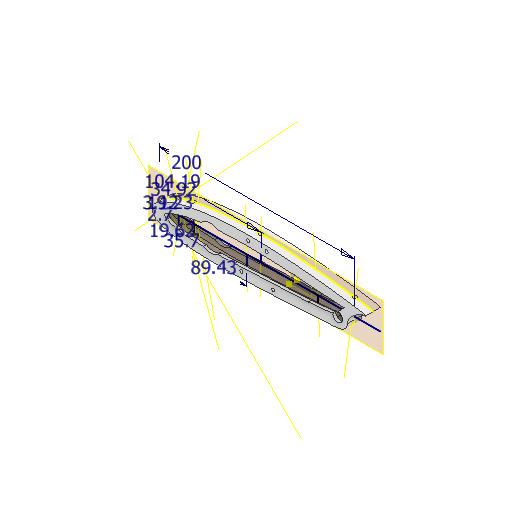
# Autodesk Inventor part: 4P.01.01.11-TW-v1-WingRibWFlapSingle
Saved by Autodesk Inventor 2025.2 (Build 292293000, 293)
## iProperties
Created: 2025-01-11
Part Number: 4P.01.01.11-TW-v1-WingRibWFlapSingle
Material: Polystyrene
Document SubType Name: Modeling
Designer: thoma
Density: 1.021 g/cm^3
Appearance: Smooth - White
Author: thoma
Autodesk Inventor part; units mm, degrees
(part 1 of 2)
ref_plane "YZ Plane" through (0, 0, 0) normal (1, 0, 0) x (0, 1, 0)
ref_plane "XZ Plane" through (0, 0, 0) normal (0, 1, 0) x (-1, 0, 0)
ref_plane "XY Plane" through (0, 0, 0) normal (0, 0, 1) x (1, 0, 0)
sketch "Sketch3" plane through (0, 0, 0) normal (0, 0, 1) x (1, 0, 0)
  line L0 (59.6953, 14.884) -> (59.6953, -12.7998) construction
  spline S0 degree 4 poles (78.1029, 11.0141) (75.5683, 12.9654) (71.7145, 13.0272) (66.8099, 13.9036) (60.7685, 14.7338) (56.2959, 15.3578) (51.7728, 15.9509) (47.2242, 16.5426) (42.6244, 17.1111) (37.9974, 17.6651) (33.3378, 18.1987) (28.6546, 18.7114) (23.9504, 19.2026) (19.2309, 19.6699) (14.5002, 20.1135) (9.7632, 20.5291) (5.025, 20.9191) (0.2903, 21.2792) (-4.4372, 21.6095) (-9.151, 21.9092) (-13.8524, 22.1766) (-18.5268, 22.4102) (-23.2002, 22.6105) (-27.8558, 22.7627) (-32.4748, 22.8704) (-37.0553, 22.9312) (-41.5904, 22.9454) (-46.0738, 22.9127) (-50.5027, 22.8323) (-54.8678, 22.7052) (-59.1755, 22.5324) (-63.394, 22.3084) (-67.5752, 22.0492) (-71.5451, 21.7209) (-75.7777, 21.4072) (-79.04, 20.9063) (-83.4863, 20.5541) (-87.0067, 20.037) (-90.7113, 19.5168) (-94.2172, 18.9459) (-97.6363, 18.3426) (-100.9342, 17.7015) (-104.1216, 17.0263) (-107.1909, 16.3187) (-110.1396, 15.5797) (-112.9656, 14.8117) (-115.6652, 14.0172) (-118.2357, 13.1965) (-120.6759, 12.3541) (-122.9817, 11.4895) (-125.1529, 10.6071) (-127.1857, 9.7065) (-129.0794, 8.7914) (-130.8324, 7.8633) (-132.4429, 6.923) (-133.9096, 5.9737) (-135.2322, 5.016) (-136.4083, 4.0508) (-137.4392, 3.0816) (-138.3215, 2.1025) (-139.0592, 1.1321) (-139.6407, 0.1249) (-140.106, -0.8362) (-140.3589, -2.0477) (-140.602, -2.598) (-140.1166, -5.4607) (-140.0539, -5.4622) (-139.4639, -6.7645) (-138.8842, -7.4979) (-138.1173, -8.3934) (-137.2199, -9.1877) (-136.1721, -9.9852) (-134.9893, -10.738) (-133.6669, -11.4655) (-132.2091, -12.1599) (-130.6156, -12.8245) (-128.8897, -13.4579) (-127.0312, -14.0591) (-125.0439, -14.6296) (-122.9287, -15.1678) (-120.6879, -15.6738) (-118.3241, -16.1476) (-115.8396, -16.5892) (-113.2366, -16.9984) (-110.5176, -17.3742) (-107.6861, -17.7183) (-104.7439, -18.0297) (-101.6943, -18.3095) (-98.5398, -18.5568) (-95.2843, -18.7732) (-91.9297, -18.9579) (-88.48, -19.1131) (-84.9381, -19.2376) (-81.3071, -19.3341) (-77.5906, -19.4015) (-73.7915, -19.4421) (-69.9139, -19.4561) (-65.961, -19.445) (-61.9362, -19.4102) (-57.8434, -19.3518) (-53.6861, -19.2727) (-49.4679, -19.1731) (-45.1932, -19.0538) (-40.8649, -18.9183) (-36.4879, -18.766) (-32.0649, -18.5992) (-27.598, -18.4192) (-23.0941, -18.227) (-18.5434, -18.0273) (-13.9382, -17.8076) (-9.3141, -17.5719) (-4.666, -17.3195) (-0.0002, -17.052) (4.6675, -16.7728) (9.3655, -16.4759) (14.0236, -16.1832) (19.545, -15.7815) (23.3079, -15.6072) (27.1098, -15.1781) (28.8959, -15.0599) knots 0 0 0 0 0 0.024672 0.034555 0.0445 0.054495 0.064543 0.074632 0.084755 0.094911 0.105094 0.115299 0.125521 0.135755 0.145995 0.156237 0.166475 0.176705 0.186921 0.197118 0.207299 0.217463 0.227605 0.23772 0.247796 0.257824 0.267798 0.277713 0.287563 0.297345 0.307053 0.31668 0.326224 0.335555 0.344908 0.354162 0.363308 0.372467 0.381393 0.390196 0.398872 0.407415 0.41582 0.424082 0.432193 0.44015 0.447945 0.455574 0.46303 0.470307 0.477401 0.484305 0.491015 0.497525 0.503831 0.509931 0.515822 0.521506 0.526986 0.53227 0.537373 0.542316 0.547131 0.552525 0.557529 0.562533 0.567581 0.57205 0.576988 0.582082 0.587354 0.592817 0.598478 0.604341 0.610406 0.616671 0.623133 0.629789 0.636632 0.643658 0.650861 0.658236 0.665777 0.673478 0.681333 0.689338 0.697486 0.705771 0.71419 0.722736 0.731403 0.740188 0.749084 0.758087 0.767192 0.776393 0.785687 0.795067 0.804529 0.814069 0.823682 0.833362 0.843106 0.852907 0.862763 0.872667 0.88262 0.892624 0.902675 0.912766 0.92289 0.933033 0.943191 0.953358 0.963531 0.973703 0.984092 1 1 1 1 1
  line L1 (159.6953, -3.8066) -> (59.6953, -3.8066) construction
  spline S1 degree 4 poles (78.1029, 11.0141) (76.6463, 11.2227) (73.9909, 10.5042) (70.2765, 8.6041) (66.0429, 5.3938) (62.3889, 1.8499) (60.314, -1.2467) (59.5572, -3.5763) (59.5773, -5.0793) knots 0 0 0 0 0 0.302475 0.43895 0.576633 0.708802 1 1 1 1 1
  spline S2 degree 4 poles (28.8959, -15.0599) (34.0984, -14.7105) (49.269, -14.182) (58.5645, -15.239) (59.5773, -5.0793) knots 0 0 0 0 0 1 1 1 1 1
  line L2 (28.8959, -15.0599) -> (34.0984, -14.7105) construction
  line L3 (34.0984, -14.7105) -> (49.269, -14.182) construction
  line L4 (49.269, -14.182) -> (58.5645, -15.239) construction
  line L5 (58.5645, -15.239) -> (59.5773, -5.0793) construction
  line L6 (78.1029, 11.0141) -> (75.5683, 12.9654) construction
  line L7 (75.5683, 12.9654) -> (71.7145, 13.0272) construction
  line L8 (71.7145, 13.0272) -> (66.8099, 13.9036) construction
  line L9 (66.8099, 13.9036) -> (60.7685, 14.7338) construction
  line L10 (60.7685, 14.7338) -> (56.2959, 15.3578) construction
  line L11 (56.2959, 15.3578) -> (51.7728, 15.9509) construction
  line L12 (51.7728, 15.9509) -> (47.2242, 16.5426) construction
  line L13 (47.2242, 16.5426) -> (42.6244, 17.1111) construction
  line L14 (42.6244, 17.1111) -> (37.9974, 17.6651) construction
  line L15 (37.9974, 17.6651) -> (33.3378, 18.1987) construction
  line L16 (33.3378, 18.1987) -> (28.6546, 18.7114) construction
  line L17 (28.6546, 18.7114) -> (23.9504, 19.2026) construction
  line L18 (23.9504, 19.2026) -> (19.2309, 19.6699) construction
  line L19 (19.2309, 19.6699) -> (14.5002, 20.1135) construction
  line L20 (14.5002, 20.1135) -> (9.7632, 20.5291) construction
  line L21 (9.7632, 20.5291) -> (5.025, 20.9191) construction
  line L22 (5.025, 20.9191) -> (0.2903, 21.2792) construction
  line L23 (0.2903, 21.2792) -> (-4.4372, 21.6095) construction
  line L24 (-4.4372, 21.6095) -> (-9.151, 21.9092) construction
  line L25 (-9.151, 21.9092) -> (-13.8524, 22.1766) construction
  line L26 (-13.8524, 22.1766) -> (-18.5268, 22.4102) construction
  line L27 (-18.5268, 22.4102) -> (-23.2002, 22.6105) construction
  line L28 (-23.2002, 22.6105) -> (-27.8558, 22.7627) construction
  line L29 (-27.8558, 22.7627) -> (-32.4748, 22.8704) construction
  line L30 (-32.4748, 22.8704) -> (-37.0553, 22.9312) construction
  line L31 (-37.0553, 22.9312) -> (-41.5904, 22.9454) construction
  line L32 (-41.5904, 22.9454) -> (-46.0738, 22.9127) construction
  line L33 (-46.0738, 22.9127) -> (-50.5027, 22.8323) construction
  line L34 (-50.5027, 22.8323) -> (-54.8678, 22.7052) construction
  line L35 (-54.8678, 22.7052) -> (-59.1755, 22.5324) construction
  line L36 (-59.1755, 22.5324) -> (-63.394, 22.3084) construction
  line L37 (-63.394, 22.3084) -> (-67.5752, 22.0492) construction
  line L38 (-67.5752, 22.0492) -> (-71.5451, 21.7209) construction
  line L39 (-71.5451, 21.7209) -> (-75.7777, 21.4072) construction
  line L40 (-75.7777, 21.4072) -> (-79.04, 20.9063) construction
  line L41 (-79.04, 20.9063) -> (-83.4863, 20.5541) construction
  line L42 (-83.4863, 20.5541) -> (-87.0067, 20.037) construction
  line L43 (-87.0067, 20.037) -> (-90.7113, 19.5168) construction
  line L44 (-90.7113, 19.5168) -> (-94.2172, 18.9459) construction
  line L45 (-94.2172, 18.9459) -> (-97.6363, 18.3426) construction
  line L46 (-97.6363, 18.3426) -> (-100.9342, 17.7015) construction
  line L47 (-100.9342, 17.7015) -> (-104.1216, 17.0263) construction
  line L48 (-104.1216, 17.0263) -> (-107.1909, 16.3187) construction
  line L49 (-107.1909, 16.3187) -> (-110.1396, 15.5797) construction
  line L50 (-110.1396, 15.5797) -> (-112.9656, 14.8117) construction
  line L51 (-112.9656, 14.8117) -> (-115.6652, 14.0172) construction
  line L52 (-115.6652, 14.0172) -> (-118.2357, 13.1965) construction
  line L53 (-118.2357, 13.1965) -> (-120.6759, 12.3541) construction
  line L54 (-120.6759, 12.3541) -> (-122.9817, 11.4895) construction
  line L55 (-122.9817, 11.4895) -> (-125.1529, 10.6071) construction
  line L56 (-125.1529, 10.6071) -> (-127.1857, 9.7065) construction
  line L57 (-127.1857, 9.7065) -> (-129.0794, 8.7914) construction
  line L58 (-129.0794, 8.7914) -> (-130.8324, 7.8633) construction
  line L59 (-130.8324, 7.8633) -> (-132.4429, 6.923) construction
  line L60 (-132.4429, 6.923) -> (-133.9096, 5.9737) construction
  line L61 (-133.9096, 5.9737) -> (-135.2322, 5.016) construction
  line L62 (-135.2322, 5.016) -> (-136.4083, 4.0508) construction
  line L63 (-136.4083, 4.0508) -> (-137.4392, 3.0816) construction
  line L64 (-137.4392, 3.0816) -> (-138.3215, 2.1025) construction
  line L65 (-138.3215, 2.1025) -> (-139.0592, 1.1321) construction
  line L66 (-139.0592, 1.1321) -> (-139.6407, 0.1249) construction
  line L67 (-139.6407, 0.1249) -> (-140.106, -0.8362) construction
  line L68 (-140.106, -0.8362) -> (-140.3589, -2.0477) construction
  line L69 (-140.3589, -2.0477) -> (-140.602, -2.598) construction
  line L70 (-140.602, -2.598) -> (-140.1166, -5.4607) construction
  line L71 (-140.1166, -5.4607) -> (-140.0539, -5.4622) construction
  line L72 (-140.0539, -5.4622) -> (-139.4639, -6.7645) construction
  line L73 (-139.4639, -6.7645) -> (-138.8842, -7.4979) construction
  line L74 (-138.8842, -7.4979) -> (-138.1173, -8.3934) construction
  line L75 (-138.1173, -8.3934) -> (-137.2199, -9.1877) construction
  line L76 (-137.2199, -9.1877) -> (-136.1721, -9.9852) construction
  line L77 (-136.1721, -9.9852) -> (-134.9893, -10.738) construction
  line L78 (-134.9893, -10.738) -> (-133.6669, -11.4655) construction
  line L79 (-133.6669, -11.4655) -> (-132.2091, -12.1599) construction
  line L80 (-132.2091, -12.1599) -> (-130.6156, -12.8245) construction
  line L81 (-130.6156, -12.8245) -> (-128.8897, -13.4579) construction
  line L82 (-128.8897, -13.4579) -> (-127.0312, -14.0591) construction
  line L83 (-127.0312, -14.0591) -> (-125.0439, -14.6296) construction
  line L84 (-125.0439, -14.6296) -> (-122.9287, -15.1678) construction
  line L85 (-122.9287, -15.1678) -> (-120.6879, -15.6738) construction
  line L86 (-120.6879, -15.6738) -> (-118.3241, -16.1476) construction
  line L87 (-118.3241, -16.1476) -> (-115.8396, -16.5892) construction
  line L88 (-115.8396, -16.5892) -> (-113.2366, -16.9984) construction
  line L89 (-113.2366, -16.9984) -> (-110.5176, -17.3742) construction
  line L90 (-110.5176, -17.3742) -> (-107.6861, -17.7183) construction
  line L91 (-107.6861, -17.7183) -> (-104.7439, -18.0297) construction
  line L92 (-104.7439, -18.0297) -> (-101.6943, -18.3095) construction
  line L93 (-101.6943, -18.3095) -> (-98.5398, -18.5568) construction
  line L94 (-98.5398, -18.5568) -> (-95.2843, -18.7732) construction
  line L95 (-95.2843, -18.7732) -> (-91.9297, -18.9579) construction
  line L96 (-91.9297, -18.9579) -> (-88.48, -19.1131) construction
  line L97 (-88.48, -19.1131) -> (-84.9381, -19.2376) construction
  line L98 (-84.9381, -19.2376) -> (-81.3071, -19.3341) construction
  line L99 (-81.3071, -19.3341) -> (-77.5906, -19.4015) construction
  line L100 (-77.5906, -19.4015) -> (-73.7915, -19.4421) construction
  line L101 (-73.7915, -19.4421) -> (-69.9139, -19.4561) construction
  line L102 (-69.9139, -19.4561) -> (-65.961, -19.445) construction
  line L103 (-65.961, -19.445) -> (-61.9362, -19.4102) construction
  line L104 (-61.9362, -19.4102) -> (-57.8434, -19.3518) construction
  line L105 (-57.8434, -19.3518) -> (-53.6861, -19.2727) construction
  line L106 (-53.6861, -19.2727) -> (-49.4679, -19.1731) construction
  line L107 (-49.4679, -19.1731) -> (-45.1932, -19.0538) construction
  line L108 (-45.1932, -19.0538) -> (-40.8649, -18.9183) construction
  line L109 (-40.8649, -18.9183) -> (-36.4879, -18.766) construction
  line L110 (-36.4879, -18.766) -> (-32.0649, -18.5992) construction
  line L111 (-32.0649, -18.5992) -> (-27.598, -18.4192) construction
  line L112 (-27.598, -18.4192) -> (-23.0941, -18.227) construction
  line L113 (-23.0941, -18.227) -> (-18.5434, -18.0273) construction
  line L114 (-18.5434, -18.0273) -> (-13.9382, -17.8076) construction
  line L115 (-13.9382, -17.8076) -> (-9.3141, -17.5719) construction
  line L116 (-9.3141, -17.5719) -> (-4.666, -17.3195) construction
  line L117 (-4.666, -17.3195) -> (-0.0002, -17.052) construction
  line L118 (-0.0002, -17.052) -> (4.6675, -16.7728) construction
  line L119 (4.6675, -16.7728) -> (9.3655, -16.4759) construction
  line L120 (9.3655, -16.4759) -> (14.0236, -16.1832) construction
  line L121 (14.0236, -16.1832) -> (19.545, -15.7815) construction
  line L122 (19.545, -15.7815) -> (23.3079, -15.6072) construction
  line L123 (23.3079, -15.6072) -> (27.1098, -15.1781) construction
  line L124 (27.1098, -15.1781) -> (28.8959, -15.0599) construction
  spline S3 degree 2 poles (-105.0858, 7.2934) (-67.1463, 15.6817) (5.1275, 10.9132) knots 0 0 0 1 1 1
  spline S4 degree 1 poles (-55.7647, -9.3123) (19.5444, -5.8596) knots 0 0 1 1
  spline S5 degree 2 poles (-105.0858, 7.2934) (-120.9896, 3.0974) (-125.0439, 0.5341) knots 0 0 0 1 1 1
  spline S6 degree 2 poles (-55.7647, -9.3123) (-113.9308, -12.3922) (-125.0439, -4.6009) knots 0 0 0 1 1 1
  spline S7 degree 2 poles (-125.0439, 0.5341) (-129.8894, -1.6172) (-125.0439, -4.6009) knots 0 0 0 1 1 1
  spline S8 degree 4 poles (19.5444, -5.8596) (28.2875, -3.3108) (52.9209, -7.0257) (48.6533, 1.9889) (56.2959, 7.2934) knots 0 0 0 0 0 1 1 1 1 1
  spline S9 degree 1 poles (5.1275, 10.9132) (56.2959, 7.2934) knots 0 0 1 1
  point P0 (17.6589, 23.5628)
  point P1 (75.883, 10.8572)
  point P2 (72.8647, 9.7686)
  point P3 (69.4179, 7.8149)
  point P4 (66.0452, 5.2617)
  point P5 (63.1887, 2.4463)
  point P6 (61.1228, -0.3317)
  point P7 (59.9357, -2.8689)
  point P8 (73.8497, 12.8198)
  point P9 (69.5533, 13.4647)
  point P10 (65.1899, 14.1023)
  point P11 (60.7936, 14.7318)
  point P12 (56.3207, 15.3468)
  point P13 (51.7945, 15.947)
  point P14 (47.2398, 16.5346)
  point P15 (42.6414, 17.1053)
  point P16 (38.0104, 17.6585)
  point P17 (33.3491, 18.1925)
  point P18 (28.6632, 18.7055)
  point P19 (23.9568, 19.1966)
  point P20 (19.2348, 19.6643)
  point P21 (14.5017, 20.1074)
  point P22 (9.7623, 20.5238)
  point P23 (5.0217, 20.9132)
  point P24 (0.2844, 21.2735)
  point P25 (-4.4451, 21.6038)
  point P26 (-9.1614, 21.9032)
  point P27 (-13.86, 22.1702)
  point P28 (-18.5361, 22.4036)
  point P29 (-23.211, 22.601)
  point P30 (-27.8721, 22.754)
  point P31 (-32.4966, 22.8611)
  point P32 (-37.0797, 22.9217)
  point P33 (-41.6169, 22.9356)
  point P34 (-46.1028, 22.9023)
  point P35 (-50.5329, 22.8216)
  point P36 (-54.9021, 22.6941)
  point P37 (-59.2065, 22.5195)
  point P38 (-63.4406, 22.2977)
  point P39 (-67.6008, 22.0302)
  point P40 (-71.6806, 21.7165)
  point P41 (-75.6814, 21.3591)
  point P42 (-79.1834, 20.9458)
  point P43 (-83.4048, 20.5095)
  point P44 (-87.1309, 20.023)
  point P45 (-90.7527, 19.494)
  point P46 (-94.2725, 18.9266)
  point P47 (-97.6845, 18.3211)
  point P48 (-100.9861, 17.6791)
  point P49 (-104.1736, 17.0026)
  point P50 (-107.2438, 16.2934)
  point P51 (-110.1931, 15.553)
  point P52 (-113.0194, 14.7835)
  point P53 (-115.7191, 13.987)
  point P54 (-118.2898, 13.165)
  point P55 (-120.7294, 12.3201)
  point P56 (-123.0349, 11.454)
  point P57 (-125.2048, 10.569)
  point P58 (-127.2364, 9.6666)
  point P59 (-129.1282, 8.7491)
  point P60 (-130.8786, 7.8185)
  point P61 (-132.486, 6.8762)
  point P62 (-133.9488, 5.9245)
  point P63 (-135.2661, 4.9648)
  point P64 (-136.4363, 3.9987)
  point P65 (-137.4592, 3.0275)
  point P66 (-138.3336, 2.0531)
  point P67 (-139.0591, 1.0763)
  point P68 (-139.6352, 0.0983)
  point P69 (-140.0613, -0.8802)
  point P70 (-140.338, -1.8576)
  point P71 (-140.4646, -2.8394)
  point P72 (-140.1239, -5.2398)
  point P73 (-139.9547, -5.7022)
  point P74 (-139.492, -6.6066)
  point P75 (-138.8844, -7.4823)
  point P76 (-138.1328, -8.3292)
  point P77 (-137.2384, -9.147)
  point P78 (-136.202, -9.9355)
  point P79 (-135.0249, -10.6943)
  point P80 (-133.7085, -11.4228)
  point P81 (-132.2548, -12.1206)
  point P82 (-130.6648, -12.7879)
  point P83 (-128.941, -13.4239)
  point P84 (-127.0846, -14.0282)
  point P85 (-125.0983, -14.6009)
  point P86 (-122.9839, -15.1415)
  point P87 (-120.7435, -15.6497)
  point P88 (-118.3798, -16.1256)
  point P89 (-115.8952, -16.569)
  point P90 (-113.2918, -16.9797)
  point P91 (-110.5723, -17.3574)
  point P92 (-107.74, -17.7027)
  point P93 (-104.797, -18.0156)
  point P94 (-101.7463, -18.2964)
  point P95 (-98.5909, -18.5451)
  point P96 (-95.3341, -18.7623)
  point P97 (-91.9783, -18.9484)
  point P98 (-88.5271, -19.1041)
  point P99 (-84.9838, -19.2298)
  point P100 (-81.3514, -19.3267)
  point P101 (-77.6332, -19.3951)
  point P102 (-73.8324, -19.4362)
  point P103 (-69.9531, -19.4509)
  point P104 (-65.9985, -19.4404)
  point P105 (-61.9719, -19.4059)
  point P106 (-57.8772, -19.3483)
  point P107 (-53.718, -19.2694)
  point P108 (-49.4979, -19.1701)
  point P109 (-45.2211, -19.0516)
  point P110 (-40.8909, -18.916)
  point P111 (-36.5118, -18.7642)
  point P112 (-32.0871, -18.5977)
  point P113 (-27.6213, -18.418)
  point P114 (-23.1183, -18.2269)
  point P115 (-18.5646, -18.0247)
  point P116 (-13.9566, -17.8054)
  point P117 (-9.3252, -17.5693)
  point P118 (-4.674, -17.317)
  point P119 (-0.0078, -17.05)
  point P120 (4.6686, -16.7695)
  point P121 (9.3513, -16.477)
  point P122 (14.0352, -16.1731)
  point P123 (18.7161, -15.8596)
  point P124 (23.3889, -15.5371)
  point P125 (78.0825, 12.164)
  point P126 (159.4818, -3.8173)
  point P127 (159.2574, -3.8401)
  point P128 (158.8836, -3.8779)
  point P129 (158.3607, -3.9307)
  point P130 (157.6896, -3.9985)
  point P131 (156.8706, -4.081)
  point P132 (155.9046, -4.1779)
  point P133 (154.7931, -4.2892)
  point P134 (153.5367, -4.4143)
  point P135 (152.1372, -4.5532)
  point P136 (150.5955, -4.7056)
  point P137 (148.914, -4.8712)
  point P138 (147.0936, -5.0494)
  point P139 (145.137, -5.2399)
  point P140 (143.0457, -5.4421)
  point P141 (140.8221, -5.6563)
  point P142 (138.4686, -5.8813)
  point P143 (135.9876, -6.1174)
  point P144 (133.3815, -6.3634)
  point P145 (130.6533, -6.6196)
  point P146 (127.8054, -6.8851)
  point P147 (124.8414, -7.1596)
  point P148 (121.7634, -7.4428)
  point P149 (118.5756, -7.7341)
  point P150 (115.2804, -8.0332)
  point P151 (111.8817, -8.3395)
  point P152 (108.3828, -8.6527)
  point P153 (104.787, -8.9722)
  point P154 (101.0985, -9.2974)
  point P155 (97.3206, -9.6283)
  point P156 (93.4572, -9.9643)
  point P157 (89.5122, -10.3048)
  point P158 (85.4898, -10.6492)
  point P159 (81.3936, -10.9969)
  point P160 (77.2284, -11.3479)
  point P161 (72.9975, -11.701)
  point P162 (68.7057, -12.0556)
  point P163 (64.3572, -12.4117)
  point P164 (59.9559, -12.7678)
  point P165 (55.5069, -13.1239)
  point P166 (51.0138, -13.4788)
  point P167 (46.4817, -13.8316)
  point P168 (41.9148, -14.182)
  point P169 (35.7035, -14.3277)
  point P170 (32.6946, -14.8708)
  point P171 (82.2459, 11.5043)
  point P172 (86.3364, 10.8401)
  point P173 (90.3495, 10.1732)
  point P174 (94.2816, 9.5051)
  point P175 (98.1288, 8.837)
  point P176 (101.8872, 8.171)
  point P177 (105.5538, 7.5086)
  point P178 (109.1244, 6.8507)
  point P179 (112.596, 6.1997)
  point P180 (115.9653, 5.5565)
  point P181 (119.2287, 4.9229)
  point P182 (122.3835, 4.3007)
  point P183 (125.4264, 3.6911)
  point P184 (128.3547, 3.0956)
  point P185 (131.1654, 2.5157)
  point P186 (133.8561, 1.9532)
  point P187 (136.4244, 1.4093)
  point P188 (138.8676, 0.8855)
  point P189 (141.1833, 0.383)
  point P190 (143.3697, -0.0964)
  point P191 (145.4247, -0.5518)
  point P192 (147.3462, -0.9817)
  point P193 (149.1327, -1.3852)
  point P194 (150.7821, -1.7608)
  point P195 (152.2935, -2.1073)
  point P196 (153.6651, -2.4241)
  point P197 (154.8954, -2.7103)
  point P198 (155.9838, -2.9647)
  point P199 (156.9291, -3.187)
  dimension "d36" = 9
  dimension "d37" = 10
  dimension "d38" = 10
  dimension "d40" = 13
  dimension "d41" = 10
  dimension "d42" = 10.5
  dimension "d43" = 10
  dimension "d44" = 10
  dimension "d45" = 9.35
  dimension "d71" = 218.5675
  dimension "d72" = 195.9715
  constraints: 4 end point, 2 midpoint, 1 horizontal, 1 point on line, 1 vertical, 168 other
  measures "d36" vertical distance of point (-107.244, 16.293) point (-105.086, 7.293)
  measures "d37" vertical distance of point (-67.601, 22.03) point (-66.949, 12.03)
  measures "d38" vertical distance of point (5.022, 20.913) point (5.128, 10.913)
  measures "d40" horizontal distance of point (-140.465, -2.839) point (-127.465, -1.751)
  measures "d41" vertical distance of point (-125.098, -14.601) point (-125.044, -4.601)
  measures "d42" vertical distance of point (-129.128, 8.749) point (-127.465, -1.751)
  measures "d43" distance of point (-55.765, -19.312) point (-55.765, -9.312)
  measures "d44" vertical distance of point (18.716, -15.86) point (19.544, -5.86)
  measures "d45" horizontal distance of point (61.123, -0.332) point (51.773, 2.507)
  measures "d71" horizontal distance of L6.start point (-140.465, -2.839)
  measures "d72" horizontal distance of point (55.507, -13.124) point (-140.465, -2.839)
extrude "Extrusion3" add sketch "Sketch3" along normal blind 15
ref_plane "Work Plane6" through (0, 0, 3) normal (0, 0, -1) x (-1, 0, 0)
sketch "Sketch4" plane through (0, 0, 3) normal (0, 0, -1) x (-1, 0, 0)
  spline S0 degree 2 poles (125.0439, 0.5341) (120.9896, 3.0974) (105.0858, 7.2934) knots 0 0 0 1 1 1 projected
  spline S1 degree 2 poles (125.0439, -4.6009) (129.8894, -1.6172) (125.0439, 0.5341) knots 0 0 0 1 1 1 projected
  spline S2 degree 2 poles (55.7647, -9.3123) (113.9308, -12.3922) (125.0439, -4.6009) knots 0 0 0 1 1 1 projected
  line L0 (-19.5444, -5.8596) -> (55.7647, -9.3123) projected
  spline S3 degree 4 poles (-56.2959, 7.2934) (-48.6533, 1.9889) (-52.9209, -7.0257) (-28.2875, -3.3108) (-19.5444, -5.8596) knots 0 0 0 0 0 1 1 1 1 1 projected
  line L1 (-5.1275, 10.9132) -> (-56.2959, 7.2934) projected
  spline S4 degree 2 poles (105.0858, 7.2934) (67.1463, 15.6817) (-5.1275, 10.9132) knots 0 0 0 1 1 1 projected
  line L2 (-5.1275, 10.9132) -> (-56.2959, 7.2934) projected
  line L3 (-19.5444, -5.8596) -> (55.7647, -9.3123) projected
  line L4 (-5.1275, 10.9132) -> (-56.2959, 7.2934) projected
  line L5 (-19.5444, -5.8596) -> (55.7647, -9.3123) projected
  line L6 (-44.1582, 5.4737) -> (-44.1582, 0)
  line L7 (-44.1582, 0) -> (113.6947, -5.8596)
  line L8 (113.6947, -5.8596) -> (112.2304, 2.7368)
  line L9 (112.2304, 2.7368) -> (47.1595, 9.1033)
  line L10 (47.1595, 9.1033) -> (-44.1582, 5.4737)
  spline S5 degree 4 poles (-48.2502, 14.3529) (-26.0454, 18.2584) (18.6498, 20.4084) (59.123, 23.9702) (113.8114, 15.0394) (137.8708, 4.0936) (137.3995, -1.5614) knots 0 0 0 0 0 0.480431 0.660322 1 1 1 1 1
  spline S6 degree 3 poles (137.3995, -1.5614) (138.7235, -7.247) (134.2293, -10.5925) (107.0224, -15.0599) knots 0 0 0 0 1 1 1 1
  spline S7 degree 2 poles (107.0224, -15.0599) (61.1303, -19.1711) (-41.9483, -11.7471) knots 0 0 0 1 1 1
  spline S8 degree 2 poles (-41.9483, -11.7471) (-55.551, -11.9815) (-56.2959, -4.6009) knots 0 0 0 1 1 1
  spline S9 degree 2 poles (-56.2959, -4.6009) (-59.1188, 7.2195) (-69.1037, 10.9132) knots 0 0 0 1 1 1
  spline S10 degree 1 poles (-69.1037, 10.9132) (-48.2502, 14.3529) knots 0 0 1 1
  point P0 (0, 0)
  point P1 (35.6575, 21.0267)
  point P2 (69.6506, 20.2948)
  point P3 (107.0224, 14.3529)
  point P4 (132.9793, 4.189)
  point P5 (137.3995, -4.6008)
  point P6 (134.9689, -7.5859)
  point P7 (61.1498, -16.5031)
  point P8 (-53.6083, -9.3122)
  point P9 (-61.15, 5.4737)
  constraints: 10 end point, 3 vertical alignment, 1 vertical, 43 other
extrude "Extrusion4" cut sketch "Sketch4" against normal blind 9 contours S5 S6 S7 S8 S9 S10
sketch "Sketch5" plane through (0, 0, 15) normal (0, 0, 1) x (1, 0, 0)
  line L0 (28.9451, -15.0416) -> (34.1476, -14.6923) construction
  spline S0 degree 4 poles (28.9451, -15.0416) (34.1476, -14.6923) (49.3182, -14.1637) (58.6137, -15.2208) (59.6265, -5.0611) knots 0 0 0 0 0 1 1 1 1 1
  line L1 (34.1476, -14.6923) -> (49.3182, -14.1637) construction
  line L2 (49.3182, -14.1637) -> (58.6137, -15.2208) construction
  line L3 (58.6137, -15.2208) -> (59.6265, -5.0611) construction
  line L4 (38.0595, 3.2028) -> (38.0595, -1.6018)
  arc A0 (36.272, -3.5905) -> (38.0595, -1.6018) centre (36.0595, -1.6018) ccw
  arc A1 (38.0595, 3.2028) -> (36.272, 5.1914) centre (36.0595, 3.2028) ccw
  line L5 (59.7445, 14.9023) -> (59.7445, -12.7815) construction
  spline S1 degree 4 poles (78.1521, 11.0324) (76.6955, 11.2409) (74.0401, 10.5225) (70.3257, 8.6224) (66.0921, 5.412) (62.4381, 1.8681) (60.3632, -1.2284) (59.6064, -3.558) (59.6265, -5.0611) knots 0 0 0 0 0 0.302475 0.43895 0.576633 0.708802 1 1 1 1 1
  line L6 (159.7445, -3.7883) -> (59.7445, -3.7883) construction
  circle A2 centre (49.7445, -3.7788) radius 5
  line L7 (-80.5289, 0.8706) -> (-80.5289, 20.817) construction
  circle A3 centre (-80.5289, 0.8706) radius 13.2395
  line L8 (-53.6688, 12.5754) -> (-53.6688, -10.9745)
  arc A4 (-53.6688, -10.9745) -> (-51.4563, -12.9632) centre (-51.6688, -10.9745) ccw
  line L9 (36.272, -3.5905) -> (-51.4563, -12.9632)
  line L10 (-51.4563, 14.5641) -> (36.272, 5.1914)
  line L11 (-80.5289, 0.8706) -> (49.6017, 0.8706) construction
  spline S2 degree 4 poles (77.9906, 11.0521) (75.6175, 12.9837) (71.7637, 13.0454) (66.8591, 13.9218) (60.8177, 14.752) (56.3451, 15.3761) (51.822, 15.9692) (47.2734, 16.5609) (42.6736, 17.1294) (38.0466, 17.6833) (33.387, 18.217) (28.7038, 18.7297) (23.9996, 19.2208) (19.2801, 19.6881) (14.5494, 20.1318) (9.8124, 20.5474) (5.0742, 20.9374) (0.3395, 21.2974) (-4.388, 21.6278) (-9.1018, 21.9274) (-13.8032, 22.1948) (-18.4776, 22.4284) (-23.151, 22.6287) (-27.8066, 22.7809) (-32.4256, 22.8886) (-37.0061, 22.9494) (-41.5412, 22.9637) (-46.0246, 22.9309) (-50.4535, 22.8506) (-54.8186, 22.7235) (-59.1263, 22.5506) (-63.3448, 22.3266) (-67.526, 22.0675) (-71.4959, 21.7392) (-75.7285, 21.4255) (-78.9908, 20.9246) (-83.4371, 20.5723) (-86.9575, 20.0553) (-90.6621, 19.5351) (-94.168, 18.9641) (-97.5871, 18.3608) (-100.885, 17.7197) (-104.0724, 17.0446) (-107.1417, 16.337) (-110.0904, 15.5979) (-112.9164, 14.8299) (-115.616, 14.0355) (-118.1865, 13.2147) (-120.6267, 12.3724) (-122.9325, 11.5078) (-125.1037, 10.6253) (-127.1365, 9.7248) (-129.0302, 8.8096) (-130.7832, 7.8816) (-132.3937, 6.9413) (-133.8604, 5.992) (-135.183, 5.0343) (-136.3591, 4.069) (-137.39, 3.0999) (-138.2723, 2.1207) (-139.01, 1.1503) (-139.5915, 0.1431) (-140.0568, -0.8179) (-140.3097, -2.0294) (-140.5528, -2.5797) (-140.0674, -5.4425) (-140.0047, -5.4439) (-139.4148, -6.7462) (-138.835, -7.4797) (-138.0682, -8.3751) (-137.1707, -9.1694) (-136.1229, -9.9669) (-134.9401, -10.7198) (-133.6177, -11.4473) (-132.1599, -12.1416) (-130.5664, -12.8063) (-128.8405, -13.4396) (-126.982, -14.0408) (-124.9947, -14.6113) (-122.8795, -15.1495) (-120.6387, -15.6555) (-118.2749, -16.1293) (-115.7904, -16.5709) (-113.1874, -16.9801) (-110.4684, -17.3559) (-107.6369, -17.7) (-104.6947, -18.0114) (-101.6451, -18.2912) (-98.4906, -18.5386) (-95.2351, -18.755) (-91.8805, -18.9397) (-88.4308, -19.0948) (-84.8889, -19.2193) (-81.2579, -19.3159) (-77.5414, -19.3833) (-73.7423, -19.4239) (-69.8647, -19.4379) (-65.9118, -19.4268) (-61.887, -19.392) (-57.7942, -19.3336) (-53.6369, -19.2544) (-49.4187, -19.1548) (-45.144, -19.0356) (-40.8157, -18.9) (-36.4387, -18.7477) (-32.0157, -18.581) (-27.5488, -18.401) (-23.0449, -18.2088) (-18.4942, -18.0091) (-13.889, -17.7894) (-9.2649, -17.5537) (-4.6168, -17.3012) (0.049, -17.0337) (4.7167, -16.7545) (9.4147, -16.4577) (14.0728, -16.1649) (19.5942, -15.7632) (23.3571, -15.5889) (27.159, -15.1599) (28.9451, -15.0416) knots 0 0 0 0 0 0.024672 0.034555 0.0445 0.054495 0.064543 0.074632 0.084755 0.094911 0.105094 0.115299 0.125521 0.135755 0.145995 0.156237 0.166475 0.176705 0.186921 0.197118 0.207299 0.217463 0.227605 0.23772 0.247796 0.257824 0.267798 0.277713 0.287563 0.297345 0.307053 0.31668 0.326224 0.335555 0.344908 0.354162 0.363308 0.372467 0.381393 0.390196 0.398872 0.407415 0.41582 0.424082 0.432193 0.44015 0.447945 0.455574 0.46303 0.470307 0.477401 0.484305 0.491015 0.497525 0.503831 0.509931 0.515822 0.521506 0.526986 0.53227 0.537373 0.542316 0.547131 0.552525 0.557529 0.562533 0.567581 0.57205 0.576988 0.582082 0.587354 0.592817 0.598478 0.604341 0.610406 0.616671 0.623133 0.629789 0.636632 0.643658 0.650861 0.658236 0.665777 0.673478 0.681333 0.689338 0.697486 0.705771 0.71419 0.722736 0.731403 0.740188 0.749084 0.758087 0.767192 0.776393 0.785687 0.795067 0.804529 0.814069 0.823682 0.833362 0.843106 0.852907 0.862763 0.872667 0.88262 0.892624 0.902675 0.912766 0.92289 0.933033 0.943191 0.953358 0.963531 0.973703 0.984092 1 1 1 1 1
  arc A5 (-51.4563, 14.5641) -> (-53.6688, 12.5754) centre (-51.6688, 12.5754) ccw
  line L12 (-140.4154, -2.8211) -> (159.531, -3.799) construction
  line L13 (-132.0364, 0.6516) -> (-132.0364, -6.3484)
  line L14 (-132.0364, -6.3484) -> (-110.3324, -12.3392)
  line L15 (-110.3324, -12.3392) -> (-104.7478, -12.3392)
  line L16 (-104.7478, -12.3392) -> (-104.7478, -17.9974)
  line L17 (-132.0364, 0.6516) -> (-110.3324, 10.5712)
  line L18 (-110.3324, 10.5712) -> (-104.1244, 10.5712)
  line L19 (-104.1244, 10.5712) -> (-104.1244, 17.0209)
  line L20 (77.9906, 11.0521) -> (75.6175, 12.9837) construction
  line L21 (75.6175, 12.9837) -> (71.7637, 13.0454) construction
  line L22 (71.7637, 13.0454) -> (66.8591, 13.9218) construction
  line L23 (66.8591, 13.9218) -> (60.8177, 14.752) construction
  line L24 (60.8177, 14.752) -> (56.3451, 15.3761) construction
  line L25 (56.3451, 15.3761) -> (51.822, 15.9692) construction
  line L26 (51.822, 15.9692) -> (47.2734, 16.5609) construction
  line L27 (47.2734, 16.5609) -> (42.6736, 17.1294) construction
  line L28 (42.6736, 17.1294) -> (38.0466, 17.6833) construction
  line L29 (38.0466, 17.6833) -> (33.387, 18.217) construction
  line L30 (33.387, 18.217) -> (28.7038, 18.7297) construction
  line L31 (28.7038, 18.7297) -> (23.9996, 19.2208) construction
  line L32 (23.9996, 19.2208) -> (19.2801, 19.6881) construction
  line L33 (19.2801, 19.6881) -> (14.5494, 20.1318) construction
  line L34 (14.5494, 20.1318) -> (9.8124, 20.5474) construction
  line L35 (9.8124, 20.5474) -> (5.0742, 20.9374) construction
  line L36 (5.0742, 20.9374) -> (0.3395, 21.2974) construction
  line L37 (0.3395, 21.2974) -> (-4.388, 21.6278) construction
  line L38 (-4.388, 21.6278) -> (-9.1018, 21.9274) construction
  line L39 (-9.1018, 21.9274) -> (-13.8032, 22.1948) construction
  line L40 (-13.8032, 22.1948) -> (-18.4776, 22.4284) construction
  line L41 (-18.4776, 22.4284) -> (-23.151, 22.6287) construction
  line L42 (-23.151, 22.6287) -> (-27.8066, 22.7809) construction
  line L43 (-27.8066, 22.7809) -> (-32.4256, 22.8886) construction
  line L44 (-32.4256, 22.8886) -> (-37.0061, 22.9494) construction
  line L45 (-37.0061, 22.9494) -> (-41.5412, 22.9637) construction
  line L46 (-41.5412, 22.9637) -> (-46.0246, 22.9309) construction
  line L47 (-46.0246, 22.9309) -> (-50.4535, 22.8506) construction
  line L48 (-50.4535, 22.8506) -> (-54.8186, 22.7235) construction
  line L49 (-54.8186, 22.7235) -> (-59.1263, 22.5506) construction
  line L50 (-59.1263, 22.5506) -> (-63.3448, 22.3266) construction
  line L51 (-63.3448, 22.3266) -> (-67.526, 22.0675) construction
  line L52 (-67.526, 22.0675) -> (-71.4959, 21.7392) construction
  line L53 (-71.4959, 21.7392) -> (-75.7285, 21.4255) construction
  line L54 (-75.7285, 21.4255) -> (-78.9908, 20.9246) construction
  line L55 (-78.9908, 20.9246) -> (-83.4371, 20.5723) construction
  line L56 (-83.4371, 20.5723) -> (-86.9575, 20.0553) construction
  line L57 (-86.9575, 20.0553) -> (-90.6621, 19.5351) construction
  line L58 (-90.6621, 19.5351) -> (-94.168, 18.9641) construction
  line L59 (-94.168, 18.9641) -> (-97.5871, 18.3608) construction
  line L60 (-97.5871, 18.3608) -> (-100.885, 17.7197) construction
  line L61 (-100.885, 17.7197) -> (-104.0724, 17.0446) construction
  line L62 (-104.0724, 17.0446) -> (-107.1417, 16.337) construction
  line L63 (-107.1417, 16.337) -> (-110.0904, 15.5979) construction
  line L64 (-110.0904, 15.5979) -> (-112.9164, 14.8299) construction
  line L65 (-112.9164, 14.8299) -> (-115.616, 14.0355) construction
  line L66 (-115.616, 14.0355) -> (-118.1865, 13.2147) construction
  line L67 (-118.1865, 13.2147) -> (-120.6267, 12.3724) construction
  line L68 (-120.6267, 12.3724) -> (-122.9325, 11.5078) construction
  line L69 (-122.9325, 11.5078) -> (-125.1037, 10.6253) construction
  line L70 (-125.1037, 10.6253) -> (-127.1365, 9.7248) construction
  line L71 (-127.1365, 9.7248) -> (-129.0302, 8.8096) construction
  line L72 (-129.0302, 8.8096) -> (-130.7832, 7.8816) construction
  line L73 (-130.7832, 7.8816) -> (-132.3937, 6.9413) construction
  line L74 (-132.3937, 6.9413) -> (-133.8604, 5.992) construction
  line L75 (-133.8604, 5.992) -> (-135.183, 5.0343) construction
  line L76 (-135.183, 5.0343) -> (-136.3591, 4.069) construction
  line L77 (-136.3591, 4.069) -> (-137.39, 3.0999) construction
  line L78 (-137.39, 3.0999) -> (-138.2723, 2.1207) construction
  line L79 (-138.2723, 2.1207) -> (-139.01, 1.1503) construction
  line L80 (-139.01, 1.1503) -> (-139.5915, 0.1431) construction
  line L81 (-139.5915, 0.1431) -> (-140.0568, -0.8179) construction
  line L82 (-140.0568, -0.8179) -> (-140.3097, -2.0294) construction
  line L83 (-140.3097, -2.0294) -> (-140.5528, -2.5797) construction
  line L84 (-140.5528, -2.5797) -> (-140.0674, -5.4425) construction
  line L85 (-140.0674, -5.4425) -> (-140.0047, -5.4439) construction
  line L86 (-140.0047, -5.4439) -> (-139.4148, -6.7462) construction
  line L87 (-139.4148, -6.7462) -> (-138.835, -7.4797) construction
  line L88 (-138.835, -7.4797) -> (-138.0682, -8.3751) construction
  line L89 (-138.0682, -8.3751) -> (-137.1707, -9.1694) construction
  line L90 (-137.1707, -9.1694) -> (-136.1229, -9.9669) construction
  line L91 (-136.1229, -9.9669) -> (-134.9401, -10.7198) construction
  line L92 (-134.9401, -10.7198) -> (-133.6177, -11.4473) construction
  line L93 (-133.6177, -11.4473) -> (-132.1599, -12.1416) construction
  line L94 (-132.1599, -12.1416) -> (-130.5664, -12.8063) construction
  line L95 (-130.5664, -12.8063) -> (-128.8405, -13.4396) construction
  line L96 (-128.8405, -13.4396) -> (-126.982, -14.0408) construction
  line L97 (-126.982, -14.0408) -> (-124.9947, -14.6113) construction
  line L98 (-124.9947, -14.6113) -> (-122.8795, -15.1495) construction
  line L99 (-122.8795, -15.1495) -> (-120.6387, -15.6555) construction
  line L100 (-120.6387, -15.6555) -> (-118.2749, -16.1293) construction
  line L101 (-118.2749, -16.1293) -> (-115.7904, -16.5709) construction
  line L102 (-115.7904, -16.5709) -> (-113.1874, -16.9801) construction
  line L103 (-113.1874, -16.9801) -> (-110.4684, -17.3559) construction
  line L104 (-110.4684, -17.3559) -> (-107.6369, -17.7) construction
  line L105 (-107.6369, -17.7) -> (-104.6947, -18.0114) construction
  line L106 (-104.6947, -18.0114) -> (-101.6451, -18.2912) construction
  line L107 (-101.6451, -18.2912) -> (-98.4906, -18.5386) construction
  line L108 (-98.4906, -18.5386) -> (-95.2351, -18.755) construction
  line L109 (-95.2351, -18.755) -> (-91.8805, -18.9397) construction
  line L110 (-91.8805, -18.9397) -> (-88.4308, -19.0948) construction
  line L111 (-88.4308, -19.0948) -> (-84.8889, -19.2193) construction
  line L112 (-84.8889, -19.2193) -> (-81.2579, -19.3159) construction
  line L113 (-81.2579, -19.3159) -> (-77.5414, -19.3833) construction
  line L114 (-77.5414, -19.3833) -> (-73.7423, -19.4239) construction
  line L115 (-73.7423, -19.4239) -> (-69.8647, -19.4379) construction
  line L116 (-69.8647, -19.4379) -> (-65.9118, -19.4268) construction
  line L117 (-65.9118, -19.4268) -> (-61.887, -19.392) construction
  line L118 (-61.887, -19.392) -> (-57.7942, -19.3336) construction
  line L119 (-57.7942, -19.3336) -> (-53.6369, -19.2544) construction
  line L120 (-53.6369, -19.2544) -> (-49.4187, -19.1548) construction
  line L121 (-49.4187, -19.1548) -> (-45.144, -19.0356) construction
  line L122 (-45.144, -19.0356) -> (-40.8157, -18.9) construction
  line L123 (-40.8157, -18.9) -> (-36.4387, -18.7477) construction
  line L124 (-36.4387, -18.7477) -> (-32.0157, -18.581) construction
  line L125 (-32.0157, -18.581) -> (-27.5488, -18.401) construction
  line L126 (-27.5488, -18.401) -> (-23.0449, -18.2088) construction
  line L127 (-23.0449, -18.2088) -> (-18.4942, -18.0091) construction
  line L128 (-18.4942, -18.0091) -> (-13.889, -17.7894) construction
  line L129 (-13.889, -17.7894) -> (-9.2649, -17.5537) construction
  line L130 (-9.2649, -17.5537) -> (-4.6168, -17.3012) construction
  line L131 (-4.6168, -17.3012) -> (0.049, -17.0337) construction
  line L132 (0.049, -17.0337) -> (4.7167, -16.7545) construction
  line L133 (4.7167, -16.7545) -> (9.4147, -16.4577) construction
  line L134 (9.4147, -16.4577) -> (14.0728, -16.1649) construction
  line L135 (14.0728, -16.1649) -> (19.5942, -15.7632) construction
  line L136 (19.5942, -15.7632) -> (23.3571, -15.5889) construction
  line L137 (23.3571, -15.5889) -> (27.159, -15.1599) construction
  line L138 (27.159, -15.1599) -> (28.9451, -15.0416) construction
  line L139 (78.1521, 11.0324) -> (76.6955, 11.2409) construction
  line L140 (76.6955, 11.2409) -> (74.0401, 10.5225) construction
  line L141 (74.0401, 10.5225) -> (70.3257, 8.6224) construction
  line L142 (70.3257, 8.6224) -> (66.0921, 5.412) construction
  line L143 (66.0921, 5.412) -> (62.4381, 1.8681) construction
  line L144 (62.4381, 1.8681) -> (60.3632, -1.2284) construction
  line L145 (60.3632, -1.2284) -> (59.6064, -3.558) construction
  line L146 (59.6064, -3.558) -> (59.6265, -5.0611) construction
  point P0 (0, 0)
  point P1 (0.0492, 0.0183)
  point P2 (78.0107, 11.05)
  point P3 (17.7081, 23.581)
  point P4 (73.8985, 12.8363)
  point P5 (69.6025, 13.483)
  point P6 (65.2391, 14.1205)
  point P7 (60.8428, 14.75)
  point P8 (56.3699, 15.3651)
  point P9 (51.8437, 15.9652)
  point P10 (47.289, 16.5528)
  point P11 (42.6906, 17.1235)
  point P12 (38.0596, 17.6768)
  point P13 (33.3983, 18.2108)
  point P14 (28.7124, 18.7238)
  point P15 (24.006, 19.2149)
  point P16 (19.284, 19.6826)
  point P17 (14.5509, 20.1257)
  point P18 (9.8115, 20.5421)
  point P19 (5.0709, 20.9315)
  point P20 (0.3336, 21.2918)
  point P21 (-4.3959, 21.6221)
  point P22 (-9.1122, 21.9215)
  point P23 (-13.8108, 22.1885)
  point P24 (-18.4869, 22.4219)
  point P25 (-23.1618, 22.6193)
  point P26 (-27.8229, 22.7723)
  point P27 (-32.4474, 22.8794)
  point P28 (-37.0305, 22.94)
  point P29 (-41.5677, 22.9538)
  point P30 (-46.0536, 22.9205)
  point P31 (-50.4837, 22.8398)
  point P32 (-49.2183, 6.3899)
  point P33 (-53.5227, 6.2154)
  point P34 (-63.3914, 22.316)
  point P35 (-67.5516, 22.0485)
  point P36 (-71.6314, 21.7347)
  point P37 (-75.6323, 21.3774)
  point P38 (-79.1342, 20.9641)
  point P39 (-83.3556, 20.5278)
  point P40 (-87.0818, 20.0413)
  point P41 (-90.7035, 19.5123)
  point P42 (-94.2233, 18.9448)
  point P43 (-97.6353, 18.3394)
  point P44 (-100.9369, 17.6974)
  point P45 (-107.1946, 16.3117)
  point P46 (-110.1439, 15.5712)
  point P47 (-112.9702, 14.8017)
  point P48 (-115.6699, 14.0052)
  point P49 (-118.2406, 13.1832)
  point P50 (-120.6802, 12.3384)
  point P51 (-122.9857, 11.4723)
  point P52 (-125.1556, 10.5873)
  point P53 (-127.1872, 9.6848)
  point P54 (-129.079, 8.7674)
  point P55 (-130.8294, 7.8368)
  point P56 (-132.4368, 6.8944)
  point P57 (-133.8996, 5.9428)
  point P58 (-135.2169, 4.983)
  point P59 (-136.3871, 4.017)
  point P60 (-137.41, 3.0458)
  point P61 (-138.2844, 2.0713)
  point P62 (-139.0099, 1.0945)
  point P63 (-139.586, 0.1165)
  point P64 (-140.0121, -0.862)
  point P65 (-140.2888, -1.8394)
  point P66 (-140.0747, -5.2215)
  point P67 (-139.9055, -5.6839)
  point P68 (-139.4428, -6.5883)
  point P69 (-138.8352, -7.464)
  point P70 (-138.0836, -8.3109)
  point P71 (-137.1892, -9.1288)
  point P72 (-136.1528, -9.9173)
  point P73 (-134.9757, -10.676)
  point P74 (-133.6593, -11.4045)
  point P75 (-132.2056, -12.1024)
  point P76 (-130.6156, -12.7696)
  point P77 (-128.8918, -13.4057)
  point P78 (-127.0354, -14.0099)
  point P79 (-125.0491, -14.5826)
  point P80 (-122.9347, -15.1233)
  point P81 (-120.6943, -15.6315)
  point P82 (-118.3306, -16.1073)
  point P83 (-115.846, -16.5507)
  point P84 (-113.2426, -16.9614)
  point P85 (-110.5231, -17.3392)
  point P86 (-107.6908, -17.6845)
  point P87 (-101.6971, -18.2782)
  point P88 (-98.5417, -18.5269)
  point P89 (-95.2849, -18.7441)
  point P90 (-91.9291, -18.9301)
  point P91 (-88.4779, -19.0858)
  point P92 (-84.9346, -19.2115)
  point P93 (-81.3022, -19.3084)
  point P94 (-77.584, -19.3768)
  point P95 (-73.7833, -19.4179)
  point P96 (-69.9039, -19.4326)
  point P97 (-65.9493, -19.4221)
  point P98 (-61.9227, -19.3876)
  point P99 (-57.828, -19.33)
  point P100 (-53.6688, -19.2511)
  point P101 (-49.4487, -19.1518)
  point P102 (-45.1719, -19.0333)
  point P103 (-40.8417, -18.8977)
  point P104 (-36.4626, -18.7459)
  point P105 (-32.0379, -18.5794)
  point P106 (-27.5721, -18.3997)
  point P107 (-23.0691, -18.2086)
  point P108 (-18.5154, -18.0064)
  point P109 (-13.9074, -17.7871)
  point P110 (-9.276, -17.551)
  point P111 (-4.6248, -17.2987)
  point P112 (0.0414, -17.0317)
  point P113 (4.7178, -16.7512)
  point P114 (9.4005, -16.4587)
  point P115 (14.0844, -16.1548)
  point P116 (18.7653, -15.8413)
  point P117 (23.4381, -15.5188)
  point P118 (159.5328, -3.7741)
  point P119 (159.3132, -3.7216)
  point P120 (158.9478, -3.6346)
  point P121 (158.4363, -3.5134)
  point P122 (157.7799, -3.3577)
  point P123 (156.9783, -3.1687)
  point P124 (156.033, -2.9464)
  point P125 (154.9446, -2.692)
  point P126 (153.7143, -2.4058)
  point P127 (152.3427, -2.089)
  point P128 (150.8313, -1.7425)
  point P129 (149.1819, -1.3669)
  point P130 (147.3954, -0.9634)
  point P131 (145.4739, -0.5335)
  point P132 (143.4189, -0.0781)
  point P133 (141.2325, 0.4013)
  point P134 (138.9168, 0.9038)
  point P135 (136.4736, 1.4276)
  point P136 (133.9053, 1.9715)
  point P137 (131.2146, 2.534)
  point P138 (128.4039, 3.1139)
  point P139 (125.4756, 3.7094)
  point P140 (122.4327, 4.319)
  point P141 (119.2779, 4.9412)
  point P142 (116.0145, 5.5748)
  point P143 (112.6452, 6.218)
  point P144 (109.1736, 6.869)
  point P145 (105.603, 7.5269)
  point P146 (101.9364, 8.1893)
  point P147 (98.178, 8.8553)
  point P148 (94.3308, 9.5234)
  point P149 (90.3987, 10.1915)
  point P150 (86.3856, 10.8584)
  point P151 (82.2951, 11.5226)
  point P152 (32.7438, -14.8525)
  point P153 (41.3873, -30.6318)
  point P154 (47.5986, -30.4861)
  point P155 (46.5309, -13.8133)
  point P156 (51.063, -13.4605)
  point P157 (55.5561, -13.1056)
  point P158 (60.0051, -12.7495)
  point P159 (64.4064, -12.3934)
  point P160 (68.7549, -12.0373)
  point P161 (73.0467, -11.6827)
  point P162 (77.2776, -11.3296)
  point P163 (81.4428, -10.9786)
  point P164 (85.539, -10.6309)
  point P165 (89.5614, -10.2865)
  point P166 (93.5064, -9.946)
  point P167 (97.3698, -9.61)
  point P168 (101.1477, -9.2791)
  point P169 (104.8362, -8.9539)
  point P170 (108.432, -8.6344)
  point P171 (111.9309, -8.3212)
  point P172 (115.3296, -8.0149)
  point P173 (118.6248, -7.7158)
  point P174 (121.8126, -7.4245)
  point P175 (124.8906, -7.1413)
  point P176 (127.8546, -6.8668)
  point P177 (130.7025, -6.6013)
  point P178 (133.4307, -6.3451)
  point P179 (136.0368, -6.0991)
  point P180 (138.5178, -5.863)
  point P181 (140.8713, -5.638)
  point P182 (143.0949, -5.4238)
  point P183 (145.1862, -5.2216)
  point P184 (147.1428, -5.0311)
  point P185 (148.9632, -4.8529)
  point P186 (150.6447, -4.6873)
  point P187 (152.1864, -4.5349)
  point P188 (153.5859, -4.396)
  point P189 (154.8423, -4.2709)
  point P190 (155.9538, -4.1596)
  point P191 (156.9198, -4.0627)
  point P192 (157.7388, -3.9802)
  point P193 (158.4099, -3.9124)
  point P194 (158.9328, -3.8596)
  point P195 (159.3066, -3.8218)
  point P196 (-132.0364, -2.8484)
  point P197 (-140.4124, -2.8212)
  point P198 (-139.5124, -2.8241)
  point P199 (-138.7234, -2.8267)
  dimension "d52" = 26.479
  dimension "d53" = 10
  dimension "d54" = 110
  dimension "d55" = 100
  dimension "d56" = 2
  dimension "d57" = 4.6493
  dimension "d58" = 7
  dimension "d59" = 3.5
  dimension "d60" = 8.379
  dimension "d61" = 30.083
  dimension "d62" = 5
  dimension "d63" = 5
  dimension "d64" = 59.8865
  dimension "d67" = 0.003
  dimension "d68" = 0.903
  dimension "d69" = 1.692
  constraints: 32 end point, 8 point on circle, 8 tangent, 6 centre point, 5 point on line, 5 vertical, 3 equal radius, 3 horizontal, 3 perpendicular, 1 midpoint, 129 other
  measures "d52" diameter of A3
  measures "d53" diameter of A2
  measures "d54" distance of L6.start A2.centre
  measures "d55" distance of L6.start L6.end
  measures "d56" radius of A5
  measures "d57" vertical distance of A2.centre L11.start
  measures "d58" distance of L14.start L17.start
  measures "d59" distance from line of L12 L17.start
  measures "d60" horizontal distance of point (-132.036, -2.848) L12.start
  measures "d61" horizontal distance of L14.end L12.start
  measures "d62" vertical distance of point (-110.144, 15.571) L17.end
  measures "d63" vertical distance of point (-110.523, -17.339) L14.end
  measures "d64" horizontal distance of L12.start L11.start
  measures "d67" distance of point (-140.412, -2.821) L12.start
  measures "d68" distance of L12.start point (-139.512, -2.824)
  measures "d69" distance of L12.start point (-138.723, -2.827)
sketch "Sketch6" plane through (0, 0, 15) normal (0, 0, 1) x (1, 0, 0)
  point P0 (0, 0)
ref_plane "Work Plane8" through (0, 0, 7.5) normal (0, 0, 1) x (1, 0, 0)
sketch "Sketch7" plane through (0, 0, 7.5) normal (0, 0, 1) x (1, 0, 0)
  line L0 (-140.4607, -2.5398) -> (86.0739, -2.5398)
  line L1 (-137.3407, -2.5398) -> (-137.3407, 3.148)
  line L2 (-137.7607, -2.5398) -> (-137.7607, -8.6916)
  line L3 (-121.2307, 12.1377) -> (-121.2307, -2.5398)
  line L4 (-105.5407, 16.6942) -> (-105.5407, -2.5398)
  line L5 (-36.2707, 22.9144) -> (-36.2707, -2.5398)
  line L6 (59.5393, 14.9056) -> (59.5393, -2.5398)
  line L7 (-120.8407, -2.5398) -> (-120.8407, -15.6289)
  line L8 (-104.7607, -2.5398) -> (-104.7607, -18.0192)
  line L9 (-51.0307, -2.5398) -> (-51.0307, -19.2083)
  line L10 (22.2132, -15.6289) -> (22.2132, -2.5398)
  point P0 (0, 0)
  point P1 (-105.5407, 7.0772)
  point P2 (-36.2707, 10.1873)
  point P3 (59.5393, 6.1829)
  dimension "d85" = 3.12
  dimension "d86" = 2.7
  dimension "d87" = 19.23
  dimension "d91" = 34.92
  dimension "d92" = 104.19
  dimension "d93" = 200
  dimension "d94" = 19.62
  dimension "d95" = 35.7
  dimension "d96" = 89.43
  constraints: 20 end point, 8 vertical, 3 midpoint, 2 parallel, 26 other
  measures "d85" distance from line of L1 point (-140.461, -2.54)
  measures "d86" distance from line of L2 point (-140.461, -2.54)
  measures "d87" distance from line of L3 point (-140.461, -2.54)
  measures "d91" horizontal distance of point (-140.461, -2.54) point (-105.541, 7.077)
  measures "d92" horizontal distance of point (-140.461, -2.54) point (-36.271, 10.187)
  measures "d93" horizontal distance of point (-140.461, -2.54) point (59.539, 6.183)
  measures "d94" distance from line of L7 point (-140.461, -2.54)
  measures "d95" distance from line of L8 point (-140.461, -2.54)
  measures "d96" distance from line of L9 point (-140.461, -2.54)
hole "Hole2" at (-137.3407, 3.148, 7.5) direction (0.7094443, -0.7047615, 0) diameter 4 depth 10 tip angle 118
hole "Hole3" at (-121.2307, 12.1377, 7.5) direction (0.3445307, -0.938775, 0) diameter 4 depth 10 tip angle 118
hole "Hole4" at (-105.5407, 16.6942, 7.5) direction (0.2240063, -0.9745877, 0) diameter 4 depth 10 tip angle 118
hole "Hole5" at (-36.2707, 22.9144, 7.5) direction (-0.0099561, -0.9999504, 0) diameter 4 depth 10 tip angle 118
hole "Hole6" at (59.5393, 14.9056, 7.5) direction (-0.1369879, -0.9905727, 0) diameter 4 depth 10 tip angle 118
hole "Hole7" at (-137.7607, -8.6916, 7.5) direction (0.6791963, 0.7339567, 0) diameter 4 depth 10 tip angle 118
hole "Hole8" at (-120.8407, -15.6289, 7.5) direction (0.2099811, 0.9777055, 0) diameter 4 depth 10 tip angle 118
hole "Hole9" at (-104.7607, -18.0192, 7.5) direction (0.0983785, 0.9951491, 0) diameter 4 depth 10 tip angle 118
hole "Hole10" at (-51.0307, -19.2083, 7.5) direction (-0.0241419, 0.9997085, 0) diameter 4 depth 10 tip angle 118
hole "Hole12" at (22.2132, -15.6289, 7.5) direction (-0.073682, 0.9972818, 0) diameter 4 depth 10 tip angle 118
extrude "Extrusion6" cut sketch "Sketch5" against normal blind 35.7 contours A2 | A3